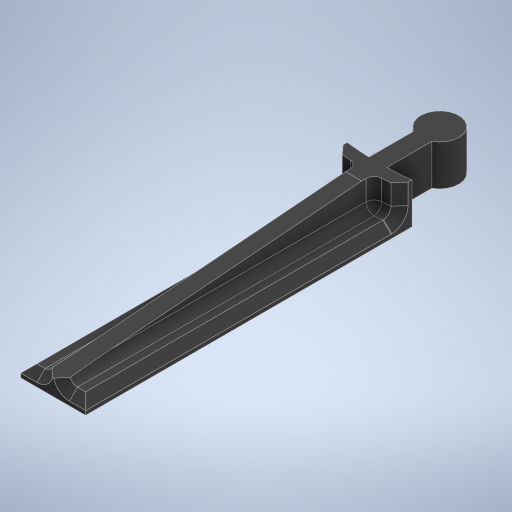
# Autodesk Inventor part: Base_2Leg
Saved by Autodesk Inventor 2023 (Build 270158000, 158)
## iProperties
Created: 2024-07-31
Part Number: Base_2Leg
Material: Generic
Document SubType Name: Modeling
Designer: Swoby
Density: 1 g/cm^3
Appearance: Default
Author: Swoby
Autodesk Inventor part; units mm, degrees
ref_plane "YZ Plane" through (0, 0, 0) normal (1, 0, 0) x (0, 1, 0)
ref_plane "XZ Plane" through (0, 0, 0) normal (0, 1, 0) x (-1, 0, 0)
ref_plane "XY Plane" through (0, 0, 0) normal (0, 0, 1) x (1, 0, 0)
sketch "Sketch1" plane through (0, 0, 0) normal (0, 1, 0) x (-1, 0, 0)
  circle A0 centre (0, 0) radius 4.7
  line L0 (2.2, 4.1533) -> (2.2, 15.2636)
  line L1 (-2.2, 15.2636) -> (-2.2, 4.1533)
  arc A1 (8, 14.817) -> (-8, 14.817) centre (0, -51.2) ccw
  line L2 (0, 15.3) -> (0, 0) construction
  line L3 (0, 15.3) -> (0, 95.3) construction
  line L4 (0, 95.3) -> (8, 95.3)
  line L5 (8, 95.3) -> (8, 14.817)
  line L6 (0, 95.3) -> (-8, 95.3)
  line L7 (0, 95.3) -> (8, 95.3) construction
  line L8 (-8, 95.3) -> (-8, 14.817)
  dimension "d0" = 9.4
  dimension "d2" = 66.5
  dimension "d4" = 2.2
  dimension "d5" = 15.3
  dimension "d6" = 2.2
  dimension "d7" = 80
  dimension "d8" = 8
  dimension "d9" = 8
  dimension "d10" = 180
  dimension "d12" = 16
  constraints: 18 end point, 7 point on circle, 3 perpendicular, 3 vertical, 2 centre point, 2 horizontal, 1 coincident, 1 collinear
  measures "d0" diameter of A0
  measures "d2" radius of A1
  measures "d4" distance between parallel lines of L2 L0
  measures "d5" distance of L2.start L2.end
  measures "d6" distance between parallel lines of L1 L2
  measures "d7" distance of L2.start L3.end
  measures "d8" distance of L3.end L4.end
  measures "d9" distance of L3.end L6.end
  measures "d10" angle of L6 L7
  measures "d12" distance of L8.end L5.end
extrude "Extrusion1" add sketch "Sketch1" along normal blind 10
sketch "Sketch2" plane through (0, 10, 0) normal (0, 1, 0) x (1, 0, 0)
  arc A0 (2.2, -15.2636) -> (8, -14.817) centre (0, 51.2) ccw projected
  line L0 (2.2, -15.2636) -> (2.2, -4.1533) projected
  arc A1 (2.2, -4.1533) -> (-2.2, -4.1533) centre (0, 0) ccw projected
  line L1 (-2.2, -4.1533) -> (-2.2, -15.2636) projected
  arc A2 (-8, -14.817) -> (-2.2, -15.2636) centre (0, 51.2) ccw projected
  line L2 (-8, -14.817) -> (-8, -95.3) projected
  line L3 (-8, -95.3) -> (8, -95.3) projected
  line L4 (8, -95.3) -> (8, -14.817) projected
  arc A3 (-2.2, -15.2636) -> (2.2, -15.2636) centre (0, 51.2) ccw
  line L5 (-2, -95.3) -> (-2, -18.2699)
  line L6 (2, -95.3) -> (2, -18.2699)
  line L7 (0, -95.3) -> (0, 0)
  arc A4 (-8, -17.817) -> (8, -17.817) centre (0, 48.2) ccw
  dimension "d15" = 66.5
  dimension "d16" = 66.5
  dimension "d19" = 2
  dimension "d20" = 2
  dimension "d21" = 3
  dimension "d22" = 3
  dimension "d23" = 66.5
  constraints: 6 end point, 6 point on circle, 4 point on line, 2 centre point, 2 vertical, 1 midpoint, 1 parallel
  measures "d15" radius of A2
  measures "d16" radius of A3
  measures "d19" distance between parallel lines of L7 L5
  measures "d20" distance between parallel lines of L6 L7
  measures "d21" distance of L2.start A4.start
  measures "d22" distance of L4.end A4.end
  measures "d23" radius of A4
extrude "Extrusion2" cut sketch "Sketch2" against normal blind 7 contours L4 L3 L6 A4 | L5 L3 L2 A4
sketch "Sketch3" plane through (2, 10, 95.3) normal (1, 0, 0) x (0, 0, -1)
  line L0 (0, 0) -> (77.0301, 0) projected
  line L1 (0, -7) -> (0, 0) projected
  line L2 (0, -7) -> (77.0301, -7) projected
  line L3 (77.0301, 0) -> (77.0301, -7) projected
  line L4 (0, -6) -> (74.0301, 0)
  point P0 (95.3, -10)
  dimension "d26" = 1
  dimension "d27" = 3
  constraints: 2 end point, 2 point on line
  measures "d26" distance of L1.start L4.start
  measures "d27" distance of L4.end L0.end
extrude "Extrusion3" cut sketch "Sketch3" against normal through all contours L0 L4 L1
fillet "Fillet1" radius 2 6 edges at (2, 3, 56.785) (-2, 3, 56.785) (-2, 6.5, 18.2699) (-5.0051, 3, 18.1114) (2, 6.5, 18.2699) (5.0051, 3, 18.1114)
chamfer "Chamfer1" distance 2 angle 45 10 edges at (-6, 3, 95.3) (-3, 3.2679, 95.3) (-8, 3, 57.5656) (-8, 3.5838, 18.4091) (-8, 7.5, 17.817) (6, 3, 95.3) (3, 3.2679, 95.3) (8, 3, 57.5656) (8, 3.5838, 18.4091) (8, 7.5, 17.817)
equation "\"d16\" = d15"
equation "\"d23\" = d15"
body "Solid1"
